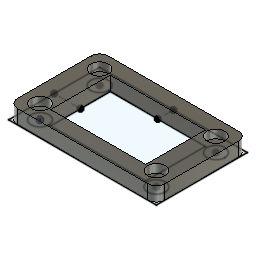
Humidity Sensor Mag Mount (Autodesk Fusion 360 design; units mm, degrees)
Autodesk Fusion 360 part; units mm, degrees
sketch "Sketch1" plane through (0, 0, 0) normal (0, 0, 1) x (1, 0, 0)
  circle A0 centre (0, 0) radius 3.1
  circle A1 centre (41, 0) radius 3.1
  circle A2 centre (0, 21) radius 3.1
  circle A3 centre (41, 21) radius 3.1
  line L0 (-5.5, 26.5) -> (46.5, 26.5)
  line L1 (46.5, 26.5) -> (46.5, -5.5)
  line L2 (46.5, -5.5) -> (-5.5, -5.5)
  line L3 (-5.5, -5.5) -> (-5.5, 26.5)
  line L4 (3.75, 21) -> (37.25, 21)
  line L5 (37.25, 21) -> (37.25, 0)
  line L6 (37.25, 0) -> (3.75, 0)
  line L7 (3.75, 0) -> (3.75, 21)
  line L8 (20.5, 26.5) -> (20.5, 21) construction
  line L9 (3.75, 10.5) -> (-5.5, 10.5) construction
  point P0 (20.5, 26.5)
  point P1 (20.5, 21)
  point P2 (-5.5, 10.5)
  point P3 (3.75, 10.5)
  dimension "d1" = 6.2
  dimension "d4" = 41
  dimension "d5" = 21
  dimension "d18" = 5.5
  dimension "d19" = 5.5
  dimension "d20" = 32
  dimension "d21" = 52
  dimension "d22" = 33.5
  dimension "d23" = 21
  constraint coincident A0.centre origin
  constraint horizontal L0
  constraint vertical L1
  constraint horizontal L2
  constraint vertical L3
  constraint horizontal L4
  constraint vertical L5
  constraint horizontal L6
  constraint vertical L7
  constraint midpoint L0 P0
  constraint midpoint L4 P1
  constraint coincident P0 L8.start
  constraint coincident P1 L8.end
  constraint midpoint L3 P2
  constraint midpoint L7 P3
  constraint coincident P3 L9.start
  constraint coincident P2 L9.end
  constraint perpendicular L0 L8
  constraint perpendicular L3 L9
  measures "d1" diameter of A0
  measures "d18" distance of A2.centre L0
  measures "d19" distance of A2.centre L3
  measures "d20" distance of L0.start L2.end
  measures "d21" distance of L0.start L0.end
  measures "d22" distance of L4.start L4.end
  measures "d23" distance of L4.start L6.end
extrude "Extrude1" add sketch "Sketch1" along normal blind 5
extrude "Extrude2" add sketch "Sketch1" along normal blind 2 contours A0 | A1 | A2 | A3
fillet "Fillet1" radius 3 4 edges at (46.5, 26.5, 2.5) (-5.5, 26.5, 2.5) (46.5, -5.5, 2.5) (-5.5, -5.5, 2.5)
